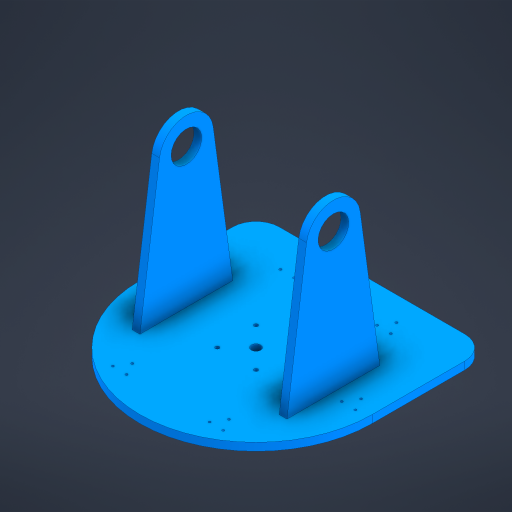
# Autodesk Inventor part: Foundation-Fork
Saved by Autodesk Inventor 2023 (Build 270158000, 158)
## iProperties
Created: 2023-09-02
Part Number: Foundation-Fork
Material: Generic
Document SubType Name: Modeling
Designer: Abhinav
Density: 1 g/cm^3
Appearance: Default(1)
Author: Abhinav
Autodesk Inventor part; units mm, degrees
ref_plane "YZ Plane" through (0, 0, 0) normal (1, 0, 0) x (0, 1, 0)
ref_plane "XZ Plane" through (0, 0, 0) normal (0, 1, 0) x (-1, 0, 0)
ref_plane "XY Plane" through (0, 0, 0) normal (0, 0, 1) x (1, 0, 0)
sketch "Sketch1" plane through (0, 0, 0) normal (1, 0, 0) x (0, 1, 0)
  circle A0 centre (0, 0) radius 19.85
  line L0 (-180, 0) -> (0, 0) construction
  line L1 (-180, 0) -> (-180, -60)
  arc A1 (4.753, -34.6758) -> (4.753, 34.6758) centre (0, 0) ccw
  line L2 (-180, -60) -> (4.753, -34.6758)
  line L3 (-180, 0) -> (-180, 60)
  line L4 (-180, 60) -> (4.753, 34.6758)
  dimension "d0" = 39.7
  dimension "d32" = 60
  dimension "d33" = 70
  dimension "d49" = 180
  constraints: 10 end point, 3 coincident, 2 centre point, 2 point on circle, 2 symmetric about line, 1 horizontal, 1 tangent, 1 vertical
  measures "d0" diameter of A0
  measures "d32" distance of L0.start L1.end
  measures "d33" diameter of A1
  measures "d49" distance of L0.start L0.end
extrude "Extrusion1" add sketch "Sketch1" along normal blind 10
ref_plane "Work Plane1" through (-180, 0, 0) normal (-1, 0, 0) x (0, 0, 1)
sketch "Sketch2" plane through (-180, 0, 0) normal (-1, 0, 0) x (0, 0, 1)
  circle A0 centre (0, 0) radius 19.85 projected
  line L0 (60, -180) -> (-60, -180) projected
  line L1 (34.6758, 4.753) -> (60, -180) projected
  arc A1 (34.6758, 4.753) -> (-34.6758, 4.753) centre (0, 0) ccw projected
  line L2 (-60, -180) -> (-34.6758, 4.753) projected
  circle A2 centre (0, 0) radius 19.85 projected
extrude "Extrusion2" add sketch "Sketch2" along normal blind 10
sketch "Sketch5" plane through (0, -180, -50) normal (0, -1, 0) x (1, 0, 0)
  arc A0 (60, 50) -> (-240, 50) centre (-90, 50) ccw
  line L0 (-90, 50) -> (35, 50) construction
  circle A1 centre (25.7561, 54.9891) radius 1.5
  circle A2 centre (35.3012, 39.5) radius 1.5
  circle A3 centre (43.9427, 55.5109) radius 1.5
  circle A4 centre (35, 50) radius 13.5 construction
  circle A5 centre (-215.3012, 39.5) radius 1.5
  circle A6 centre (-205.7561, 54.9891) radius 1.5
  circle A7 centre (-215, 50) radius 13.5 construction
  circle A8 centre (-223.9427, 55.5109) radius 1.5
  line L1 (60, 50) -> (-240, 50)
  line L2 (-240, 50) -> (-240, -100)
  line L3 (-240, -100) -> (60, -100)
  line L4 (60, -100) -> (60, 50)
  circle A9 centre (-90, 50) radius 6
  line L5 (-180, -10) -> (-180, 110) construction
  line L6 (-180, 50) -> (0, 50) construction
  line L7 (0, 110) -> (0, -10) construction
  line L8 (-90, 50) -> (-90, 90)
  line L9 (-215, 50) -> (-152.5, 158.2532) construction
  line L10 (-152.5, 158.2532) -> (-27.5, 158.2532) construction
  line L11 (-27.5, 158.2532) -> (35, 50) construction
  line L12 (35, 50) -> (-27.5, -58.2532) construction
  line L13 (-27.5, -58.2532) -> (-152.5, -58.2532) construction
  line L14 (-152.5, -58.2532) -> (-215, 50) construction
  circle A10 centre (-152.1988, -68.7532) radius 1.5
  circle A11 centre (-161.7439, -53.264) radius 1.5
  circle A12 centre (-152.5, -58.2532) radius 13.5 construction
  circle A13 centre (-143.5573, -52.7423) radius 1.5
  circle A14 centre (-27.1988, -68.7532) radius 1.5
  circle A15 centre (-36.7439, -53.264) radius 1.5
  circle A16 centre (-27.5, -58.2532) radius 13.5 construction
  circle A17 centre (-18.5573, -52.7423) radius 1.5
  circle A18 centre (-152.1988, 147.7532) radius 1.5
  circle A19 centre (-161.7439, 163.2423) radius 1.5
  circle A20 centre (-152.5, 158.2532) radius 13.5 construction
  circle A21 centre (-143.5573, 163.764) radius 1.5
  circle A22 centre (-27.1988, 147.7532) radius 1.5
  circle A23 centre (-36.7439, 163.2423) radius 1.5
  circle A24 centre (-27.5, 158.2532) radius 13.5 construction
  circle A25 centre (-18.5573, 163.764) radius 1.5
  line L15 (-65, 75) -> (-115, 75) construction
  line L16 (-115, 75) -> (-115, 25) construction
  line L17 (-115, 25) -> (-65, 25) construction
  line L18 (-65, 25) -> (-65, 75) construction
  line L19 (-65, 75) -> (-115, 25) construction
  line L20 (-115, 75) -> (-65, 25) construction
  circle A26 centre (-65, 75) radius 2.5
  circle A27 centre (-115, 75) radius 2.5
  circle A28 centre (-65, 25) radius 2.5
  circle A29 centre (-115, 25) radius 2.5
  point P0 (35, 50)
  point P1 (35, 50)
  point P2 (35, 50)
  point P3 (-215, 50)
  point P4 (-215, 50)
  point P5 (-215, 50)
  point P6 (-215, 50)
  point P7 (-152.5, -58.2532)
  point P8 (-152.5, -58.2532)
  point P9 (-152.5, -58.2532)
  point P10 (-152.5, -58.2532)
  point P11 (-27.5, -58.2532)
  point P12 (-27.5, -58.2532)
  point P13 (-27.5, -58.2532)
  point P14 (-27.5, -58.2532)
  point P15 (-152.5, 158.2532)
  point P16 (-152.5, 158.2532)
  point P17 (-152.5, 158.2532)
  point P18 (-152.5, 158.2532)
  point P19 (-27.5, 158.2532)
  point P20 (-27.5, 158.2532)
  point P21 (-27.5, 158.2532)
  point P22 (-27.5, 158.2532)
  point P23 (-90, 50)
  dimension "d21" = 300
  dimension "d25" = 125
  dimension "d30" = 12
  dimension "d34" = 40
  dimension "d35" = 150
  dimension "d36" = 50
  dimension "d37" = 50
  dimension "d38" = 5
  constraints: 38 end point, 30 centre point, 6 coincident, 4 midpoint, 4 parallel, 3 equal radius, 3 horizontal, 3 perpendicular, 2 point on circle, 1 vertical, 13 other
  measures "d21" diameter of A0
  measures "d25" distance of L0.start L0.end
  measures "d30" diameter of A9
  measures "d34" distance of L8.start L8.end
  measures "d35" distance of L1.end L2.end
  measures "d36" distance of L17.end L16.end
  measures "d37" distance of L16.end L15.end
  measures "d38" diameter of A29
extrude "Extrusion5" add sketch "Sketch5" along normal blind 10 contours L1 A9 A0 | L4 L3 L2 L1 A9
fillet "Fillet1" radius 30 2 edges at (-240, -185, -150) (60, -185, -150)
sketch "Sketch8" plane through (60, -190, 0) normal (1, 0, 0) x (0, 0, -1)
  line L0 (60, 10) -> (-60, 10) projected
  line L1 (60, 10) -> (105, 10)
  line L2 (0, 10) -> (120, 10) projected
  line L3 (105, 10) -> (105, 31) construction
  circle A0 centre (105, 31) radius 8.5527
  point P0 (0, 190)
  dimension "d44" = 45
  dimension "d45" = 21
  constraints: 4 end point, 1 centre point, 1 coincident, 1 point on line, 1 vertical
  measures "d44" distance of L0.start L1.end
  measures "d45" distance of L1.end L3.end
extrude "Extrusion7" [suppressed]
body "Solid1"
